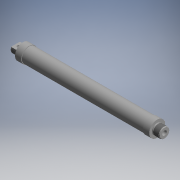
# Autodesk Inventor part: 193995 DSNU-63-500-P---(A----0-ZR)
Saved by Autodesk Inventor 2017.3 (Build 213256000, 256)
## iProperties
Part Number: 193995 DSNU-63-500-P---(A----0-ZR)
Material: Generic
Catalog Web Link: www.cadenas.de
Description: DSNU---(ZR)-Standard cylinder
Vendor: FESTO
Document SubType Name: Modeling
Designer: partserver
Manufacturer: FESTO
Mass: 465.657 g
Surface Area: 2551.46 cm^2
Volume: 465.657 cm^3
Density: 1 g/cm^3
Appearance: PSOLRGB-192-192-192
Category: PARTsolutions
Company: FESTO
Title: 193995 DSNU-63-500-P
Author: Cadenas PARTsolutions
Comments: Standard cylinder
PSOL_IDENT_0: {$CADENAS_DATA\23d-libs\festo\parts\d\dsnu\parts\dsnu_metric_zr.prj},237 {VTYP=3D},{NB=193995 DSNU-6
PSOL_IDENT_1: 3-500-P---(A----0-ZR)},{LINA=193995 DSNU-63-500-P},{NN=DSNU---(ZR)},{DATE=22.07.2021 10:44:28},{GEOM
PSOL_IDENT_2: DATE=22.07.2021 10:44:00},{VERSION=},{LINEID=100},{WBVAR=TNR,HUB,DA,PE,ZD,VS,KA,K8,KP,R8},{WBNUMERIC=
PSOL_IDENT_3: HUB,K8}  {NB=193995 DSNU-63-500-P---(A----0-ZR)},{LINA=193995 DSNU-63-500-P},{KT=DUMMY},{TNR=193995}
PSOL_IDENT_4: ,{TYP=DSNU-63},{DSNU=METRIC},{DE=D},{KDM=63},{HUB=500},{DA=P},{DA1='P','PPV','PPS'},{PE=A},{ZD=-},{V
PSOL_IDENT_5: S=-},{VSALG='-','Q'},{KA=-},{KAALG='-','S2'},{K8=0},{KP=-},{KPALG='-','KP'},{R8=-},{R81='-','R8'},{R
PSOL_IDENT_6: 8H=34.200},{A1=70},{A2=500},{A3=10},{A4=87.5},{AB=44},{AM=32},{B=45},{BB=4},{BE=M45x1,5},{BENDM=45.0
PSOL_IDENT_7: 00},{BEKDM=43.160},{BEP=1.500},{BS=11.0},{B1=72},{B2=17},{B3=44},{B4=15},{B5=36.0},{B6=18},{B7=4},{C
PSOL_IDENT_8: D=16},{D=70},{D1=45},{D2=20},{D3=65.4},{D4=16.0},{D5=66.0},{D6=60},{D7=45},{EE=G3/8},{EENDM=16.6620}
PSOL_IDENT_9: ,{EEKDM=14.9500},{EW=21},{F=52},{FF=M8},{FFNDM=8.000},{FFKDM=6.466},{F1=36},{H=72},{H1=8},{KK=M16x1.
PSOL_IDENT_10: 5},{KKNDM=16.0000},{KKKDM=13.5460},{KKP=1.500},{K1=M10},{K1NDM=10.000},{K1KDM=8.160},{K2=3.5},{KV=0}
PSOL_IDENT_11: ,{KW=10},{L=16},{LH=15.0},{LK=28.0},{L1=172.2},{L2=94.2},{L3=13.0},{L4=33.0},{L5=30},{L6=77},{L7=44}
PSOL_IDENT_12: ,{L8=28.0},{L9=32.0},{L10=117.2},{L11=132.2},{L12=94.2},{L13=184.2},{ST=11.0},{SW=17},{T=16},{WH=45}
PSOL_IDENT_13: ,{X=4.7},{XC=156.2},{K1KP=72},{K2KP=M10},{K2KPNDM=10.000},{K3KP=21},{K4KP=36.0},{K5KP=121.5},{K6KP=8
PSOL_IDENT_14: .5},{K7KP=38},{K8KP=54.0},{K9KP=24.0},{K10KP=8.0},{K11KP=32},{K12KP=G1/8},{K12KPNDM=9.728},{K13KP=86
PSOL_IDENT_15: },{ZRSTART=61},{MHL=51.000},{ZRL=38.2},{C=25.200},{WHX=15.000},{LD1=42.800},{LD2=42.800},{AD1=17.000
PSOL_IDENT_16: },{AD2=13.000},{AD3=17.000},{AD4=13.000},{AD5=13.000},{MH1=14.000},{MH2=3.100},{MH3=20.200},{KP1=48.
PSOL_IDENT_17: 000},{KP2=33.000},{KP3=25.000},{KP4=40.000},{KP5=50.000},{KPC=36.000},{KPF=3.000},{KPG=30.000},{KPH=
PSOL_IDENT_18: 115.500},{KPJ=37.500},{KPK=17.000},{KPL=6.000},{KPR3=1.500},{KPR=37.000},{KPS=28.500},{MLD1=62.000},
PSOL_IDENT_19: {MLD2=58.000},{MLD3=5.000},{MLL1=18.000},{PPVSTD=20.000},{PPVMH=43.000},{PPVMQ=8.000},{PPVY=24.200},
PSOL_IDENT_20: {PPVZ=20.500},{PPVA=5.000},{PPVB=0.500},{PPVC=0.800},{PPVD=1.500},{PPVE=11.000},{PPVH=28.200},{KL1=8
PSOL_IDENT_21: 5.2},{SWL=8.000},{K3L=10.500},{ES1=0.000},{ES2=12.000},{KPVERS=0},{HUB1=500},{NUTOFF=8.500},{DIMZJRE
PSOL_IDENT_22: AR=660.2},{KAVERS=0},{VERS=1},{H2=0}
NB: 193995 DSNU-63-500-P---(A----0-ZR)
NN: DSNU---(ZR)
NT: Standard cylinder
NBSYN: $TNR. $TYP.-$HUB1.-$DA.---($PE.$ZD.$VS.$KA.$KP.$K8.$R8.ZR)
LINA: 193995 DSNU-63-500-P
CATALOG: Festo
TNR: 193995
TYP: DSNU-63
DSNU: METRIC
DE: D
KDM: 63
HUB: 500
DA: P
DA1: 'P','PPV','PPS'
PE: A
ZD: -
VS: -
KA: -
K8: 0
KP: -
R8: -
R81: '-','R8'
R8H: 34.2
A1: 70
A2: 500
A3: 10
A4: 87.5
AB: 44
AM: 32
B: 45
BB: 4
BE: M45x1,5
BENDM: 45
BEKDM: 43.16
BEP: 1.5
BS: 11
B1: 72
B2: 17
B3: 44
B4: 15
B5: 36
B6: 18
B7: 4
CD: 16
D: 70
D1: 45
D2: 20
D3: 65.4
D4: 16
D5: 66
D6: 60
D7: 45
EE: G3/8
EENDM: 16.662
EEKDM: 14.95
EW: 21
F: 52
FF: M8
FFNDM: 8
FFKDM: 6.466
F1: 36
H: 72
H1: 8
KK: M16x1.5
KKNDM: 16
KKKDM: 13.546
KKP: 1.5
K1: M10
K1NDM: 10
K1KDM: 8.16
K2: 3.5
KV: 0
KW: 10
L: 16
LH: 15
LK: 28
L3: 13
L4: 33
L5: 30
L6: 77
L7: 44
L8: 28
L9: 32
L13: 184.2
ST: 11
SW: 17
T: 16
X: 4.7
K1KP: 72
K2KP: M10
K2KPNDM: 10
K3KP: 21
K4KP: 36
K5KP: 121.5
K6KP: 8.5
K7KP: 38
K8KP: 54
K9KP: 24
K10KP: 8
K11KP: 32
K12KP: G1/8
K12KPNDM: 9.728
K13KP: 86
MHL: 51
C: 25.2
WHX: 15
LD1: 42.8
LD2: 42.8
AD1: 17
AD2: 13
AD3: 17
AD4: 13
AD5: 13
MH1: 14
MH2: 3.1
MH3: 20.2
KP1: 48
KP2: 33
KP3: 25
KP4: 40
KP5: 50
KPC: 36
KPF: 3
KPG: 30
KPH: 115.5
KPJ: 37.5
KPK: 17
KPL: 6
KPR3: 1.5
KPR: 37
KPS: 28.5
MLD1: 62
MLD2: 58
MLD3: 5
MLL1: 18
PPVSTD: 20
PPVMH: 43
PPVMQ: 8
PPVY: 24.2
PPVZ: 20.5
PPVA: 5
PPVB: 0.5
PPVC: 0.8
PPVD: 1.5
PPVE: 11
PPVH: 28.2
SWL: 8
K3L: 10.5
ES1: 0
ES2: 12
NUTOFF: 8.5
H2: 0
SUPPLIER: FESTO
ARTICLENO: 193995 DSNU-63-500-P---(A----0-ZR)
BOMINFO: 193995 DSNU-63-500-P
CREATOR: CADENAS GmbH
Autodesk Inventor part; units mm, degrees
sketch "Sketch_22" plane through (0, 0, 0) normal (0, 0, 1) x (1, 0, 0)
  line L0 (33, 0) -> (0, 0)
  line L1 (0, 0) -> (0, 20.8)
  line L2 (0, 20.8) -> (0.6, 21.4)
  line L3 (0.6, 21.4) -> (3, 21.4)
  line L4 (3, 21.4) -> (3.6351, 22.5)
  line L5 (3.6351, 22.5) -> (27.3649, 22.5)
  line L6 (27.3649, 22.5) -> (27.8268, 21.7)
  arc A0 (27.8268, 21.7) -> (28.3464, 21.4) centre (28.3464, 22) ccw
  line L7 (28.3464, 21.4) -> (29.4, 21.4)
  arc A1 (29.4, 21.4) -> (30, 22) centre (29.4, 22) ccw
  line L8 (30, 22) -> (30, 22.5)
  line L9 (30, 22.5) -> (33, 22.5)
  line L10 (33, 22.5) -> (33, 0)
  line L11 (33, 0) -> (0, 0)
  constraints: 24 end point, 4 point on circle, 2 centre point
revolve "Revolution1" add sketch "Sketch_22" angle 360 about axis through (33, 0, 0) along (1, 0, 0)
thread "Thread1" size "M45x1.5" class "6g" standard "ISO Metric profile" full length
sketch "Sketch_2" plane through (33, 0, 0) normal (1, 0, 0) x (0, 0, -1)
  arc A0 (-12.7904, 32.5792) -> (12.7904, 32.5792) centre (0, 0) ccw
  arc A1 (12.6, 32.8585) -> (12.7904, 32.5792) centre (12.9, 32.8585) ccw
  line L0 (12.6, 32.8585) -> (12.6, 34.8)
  arc A2 (12.6, 34.8) -> (12.4, 35) centre (12.4, 34.8) ccw
  line L1 (12.4, 35) -> (-12.4, 35)
  arc A3 (-12.4, 35) -> (-12.6, 34.8) centre (-12.4, 34.8) ccw
  line L2 (-12.6, 34.8) -> (-12.6, 32.8585)
  arc A4 (-12.7904, 32.5792) -> (-12.6, 32.8585) centre (-12.9, 32.8585) ccw
  constraints: 10 point on circle, 6 end point, 5 centre point
extrude "Extrusion1" add sketch "Sketch_2" along normal blind 28
sketch "Sketch_3" plane through (0, 0, 0) normal (0, 0, 1) x (1, 0, 0)
  line L0 (599.2, 0) -> (61, 0)
  line L1 (61, 0) -> (61, 32.7)
  line L2 (61, 32.7) -> (599.2, 32.7)
  line L3 (599.2, 32.7) -> (599.2, 0)
  line L4 (599.2, 0) -> (61, 0)
  constraints: 10 end point
revolve "Revolution2" add sketch "Sketch_3" angle 360 about axis through (599.2, 0, 0) along (1, 0, 0)
sketch "Sketch_16" plane through (599.2, 0, 0) normal (1, 0, 0) x (0, 0, -1)
  arc A0 (-12.7904, 32.5792) -> (12.7904, 32.5792) centre (0, 0) ccw
  arc A1 (12.6, 32.8585) -> (12.7904, 32.5792) centre (12.9, 32.8585) ccw
  line L0 (12.6, 32.8585) -> (12.6, 34.8)
  arc A2 (12.6, 34.8) -> (12.4, 35) centre (12.4, 34.8) ccw
  line L1 (12.4, 35) -> (-12.4, 35)
  arc A3 (-12.4, 35) -> (-12.6, 34.8) centre (-12.4, 34.8) ccw
  line L2 (-12.6, 34.8) -> (-12.6, 32.8585)
  arc A4 (-12.7904, 32.5792) -> (-12.6, 32.8585) centre (-12.9, 32.8585) ccw
  constraints: 10 point on circle, 6 end point, 5 centre point
extrude "Extrusion2" add sketch "Sketch_16" along normal blind 28
sketch "Sketch_5" plane through (0, 0, 0) normal (0, 0, 1) x (1, 0, 0)
  line L0 (660.2, 0) -> (627.2, 0)
  line L1 (627.2, 0) -> (627.2, 22.5)
  line L2 (627.2, 22.5) -> (630.2, 22.5)
  line L3 (630.2, 22.5) -> (630.2, 22)
  arc A0 (630.2, 22) -> (630.8, 21.4) centre (630.8, 22) ccw
  line L4 (630.8, 21.4) -> (631.8536, 21.4)
  arc A1 (631.8536, 21.4) -> (632.3732, 21.7) centre (631.8536, 22) ccw
  line L5 (632.3732, 21.7) -> (632.8351, 22.5)
  line L6 (632.8351, 22.5) -> (656.5649, 22.5)
  line L7 (656.5649, 22.5) -> (657.2, 21.4)
  line L8 (657.2, 21.4) -> (659.6, 21.4)
  line L9 (659.6, 21.4) -> (660.2, 20.8)
  line L10 (660.2, 20.8) -> (660.2, 0)
  line L11 (660.2, 0) -> (627.2, 0)
  constraints: 24 end point, 4 point on circle, 2 centre point
revolve "Revolution3" add sketch "Sketch_5" angle 360 about axis through (660.2, 0, 0) along (1, 0, 0)
thread "Thread2" size "M45x1.5" class "6g" standard "ISO Metric profile" full length
sketch "Sketch_6" plane through (0, 0, 0) normal (0, 1, 0) x (-1, 0, 0)
  line L0 (-628.2, -31.5) -> (-628.2, -10.5)
  line L1 (-628.2, -10.5) -> (-660.2, -10.5)
  line L2 (-660.2, -10.5) -> (-660.2, 10.5)
  line L3 (-660.2, 10.5) -> (-628.2, 10.5)
  line L4 (-628.2, 10.5) -> (-628.2, 31.5)
  line L5 (-628.2, 31.5) -> (-681.2, 31.5)
  line L6 (-681.2, 31.5) -> (-681.2, -31.5)
  line L7 (-681.2, -31.5) -> (-628.2, -31.5)
  constraints: 16 end point
extrude "Extrusion3" cut sketch "Sketch_6" along normal mid plane 70
sketch "Sketch7" plane through (656.5649, -19.8997, -10.5) normal (0, 0, -1) x (-1, 0, 0)
  point P0 (12.3649, 19.8997)
hole "Hole1" at (644.2, 0, -10.5) direction (0, 0, 1) diameter 16 depth 21
sketch "Sketch8" plane through (33, 35, 12.4) normal (0, 1, 0) x (1, 0, 0)
  point P0 (13, 12.4)
hole "Hole2" at (46, 35, 0) direction (0, -1, 0) diameter 14.95 depth 17 countersink diameter 16.662 countersink angle 90 thread size "G16.662x1.337" designation "G 3/8" standard "ISO Pipe Threads"
sketch "Sketch9" plane through (599.2, 35, 12.4) normal (0, 1, 0) x (1, 0, 0)
  point P0 (15, 12.4)
hole "Hole3" at (614.2, 35, 0) direction (0, -1, 0) diameter 14.95 depth 17 countersink diameter 16.662 countersink angle 90 thread size "G16.662x1.337" designation "G 3/8" standard "ISO Pipe Threads"
sketch "Sketch_64" plane through (0, 0, 0) normal (0, 0, 1) x (1, 0, 0)
  line L0 (588.95, 0) -> (-12, 0)
  line L1 (-12, 0) -> (-12, 10)
  line L2 (-12, 10) -> (73.2, 10)
  line L3 (73.2, 10) -> (73.2, 31.5)
  line L4 (73.2, 31.5) -> (588.95, 31.5)
  line L5 (588.95, 31.5) -> (588.95, 0)
  line L6 (588.95, 0) -> (-12, 0)
  constraints: 14 end point
revolve "Revolution4" cut sketch "Sketch_64" angle 360 about axis through (588.95, 0, 0) along (1, 0, 0)
ref_plane "FDT_FRONT_XY" through (33, 0, 0) normal (1, 0, 0) x (0, 0, -1)
ref_plane "FDT_FRONT_YZ" through (33, 0, 0) normal (0, 0, -1) x (0, 1, 0)
ref_plane "FDT_FRONT_ZX" through (33, 0, 0) normal (0, 1, 0) x (1, 0, 0)
ref_plane "FDT_QSFRONT_XY" through (46, 35, 0) normal (0, 1, 0) x (0, 0, 1)
ref_plane "FDT_QSFRONT_YZ" through (46, 35, 0) normal (0, 0, 1) x (1, 0, 0)
ref_plane "FDT_QSFRONT_ZX" through (46, 35, 0) normal (1, 0, 0) x (0, 1, 0)
ref_plane "FDT_QSREAR_XY" through (614.2, 35, 0) normal (0, 1, 0) x (0, 0, 1)
ref_plane "FDT_QSREAR_YZ" through (614.2, 35, 0) normal (0, 0, 1) x (1, 0, 0)
ref_plane "FDT_QSREAR_ZX" through (614.2, 35, 0) normal (1, 0, 0) x (0, 1, 0)
ref_plane "FDT_REAR_XY" through (627.2, 0, 0) normal (-1, 0, 0) x (0, 0, -1)
ref_plane "FDT_REAR_YZ" through (627.2, 0, 0) normal (0, 0, -1) x (0, -1, 0)
ref_plane "FDT_REAR_ZX" through (627.2, 0, 0) normal (0, -1, 0) x (-1, 0, 0)
ref_plane "FDT_SMBR1_XY" through (70.5, 0, 0) normal (-1, 0, 0) x (0, 0, 1)
ref_plane "FDT_SMBR1_YZ" through (70.5, 0, 0) normal (0, 0, 1) x (0, 1, 0)
ref_plane "FDT_SMBR1_ZX" through (70.5, 0, 0) normal (0, 1, 0) x (-1, 0, 0)
ref_plane "FDT_SMBR2_XY" through (589.7, 0, 0) normal (-1, 0, 0) x (0, 0, 1)
ref_plane "FDT_SMBR2_YZ" through (589.7, 0, 0) normal (0, 0, 1) x (0, 1, 0)
ref_plane "FDT_SMBR2_ZX" through (589.7, 0, 0) normal (0, 1, 0) x (-1, 0, 0)
ref_plane "FDT_SWIVELAXIS_XY" through (644.2, 0, 0) normal (0, 0, 1) x (1, 0, 0)
ref_plane "FDT_SWIVELAXIS_YZ" through (644.2, 0, 0) normal (1, 0, 0) x (0, 1, 0)
ref_plane "FDT_SWIVELAXIS_ZX" through (644.2, 0, 0) normal (0, 1, 0) x (0, 0, 1)
ref_plane "NUT_XY" through (8.5, 0, 0) normal (1, 0, 0) x (0, 0, -1)
ref_plane "NUT_YZ" through (8.5, 0, 0) normal (0, 0, -1) x (0, 1, 0)
ref_plane "NUT_ZX" through (8.5, 0, 0) normal (0, 1, 0) x (1, 0, 0)
ref_plane "ZR_XY" through (0, 0, 0) normal (-1, 0, 0) x (0, 0, -1)
ref_plane "ZR_YZ" through (0, 0, 0) normal (0, 0, -1) x (0, -1, 0)
ref_plane "ZR_ZX" through (0, 0, 0) normal (0, -1, 0) x (-1, 0, 0)
ref_plane "ZYL_XY" through (33, 0, 0) normal (1, 0, 0) x (0, 0, -1)
ref_plane "ZYL_YZ" through (33, 0, 0) normal (0, 0, -1) x (0, 1, 0)
ref_plane "ZYL_ZX" through (33, 0, 0) normal (0, 1, 0) x (1, 0, 0)
body "Solid1"
